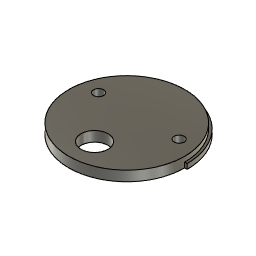
Bulkplate_InnerPayload_Cap_Subscale v1 (Autodesk Fusion 360 design; units mm, degrees)
Autodesk Fusion 360 part; units mm, degrees
sketch "Sketch1" plane through (0, 0, 0) normal (0, 0, 1) x (1, 0, 0)
  circle A0 centre (0, 0) radius 38.0746
  dimension "d1" = 76.1492
  constraint coincident A0.centre origin
  measures "d1" diameter of A0
extrude "Extrude1" add sketch "Sketch1" along normal blind 3.175
sketch "Sketch2" plane through (0, 0, 3.175) normal (0, 0, 1) x (-1, 0, 0)
  circle A0 centre (0, 0) radius 38.0746
  circle A1 centre (0, 0) radius 36.5125
  dimension "d4" = 73.025
  constraint concentric A0 A1
  measures "d4" diameter of A1
extrude "Extrude2" add sketch "Sketch2" along normal blind 3.175 contours A1
sketch "Sketch3" plane through (0, 0, 6.35) normal (0, 0, 1) x (-1, 0, 0)
  circle A0 centre (0, 0) radius 36.5125
  circle A1 centre (25.4, -7.62) radius 3.175
  circle A2 centre (-25.4, -7.62) radius 3.175
  circle A3 centre (0, 20.6756) radius 5.08
  circle A4 centre (0, 0) radius 38.0746
  dimension "d7" = 50.8
  dimension "d8" = 25.4
  dimension "d9" = 7.62
  dimension "d10" = 6.35
  dimension "d11" = 6.35
  dimension "d12" = 10.16
  dimension "d13" = 20.6756
  measures "d7" distance of A1.centre A2.centre
  measures "d8" horizontal distance of A0.centre A1.centre
  measures "d9" vertical distance of A0.centre A2.centre
  measures "d10" diameter of A2
  measures "d11" diameter of A1
  measures "d12" diameter of A3
  measures "d13" distance of A3.centre A0.centre
extrude "Extrude3" cut sketch "Sketch3" against normal blind 6.35 contours A1 | A2 | A3
sketch "Sketch4" plane through (0, 0, 6.35) normal (0, 0, 1) x (-1, 0, 0)
  circle A0 centre (-25.4, -7.62) radius 3.175
  circle A1 centre (0, 20.6756) radius 5.08
  circle A2 centre (25.4, -7.62) radius 3.175
  circle A3 centre (0, 0) radius 36.5125
  line L0 (38.0746, -0.0035) -> (36.5125, -0.0035)
  line L1 (-38.0746, 0.0019) -> (-36.5125, 0.0019)
  arc A4 (38.0746, -0.0035) -> (-38.0746, 0.0019) centre (0, 0) ccw
  arc A5 (36.5125, -0.0035) -> (-36.5125, 0.0019) centre (0, 0) ccw
  circle A6 centre (0, 20.6756) radius 8.509
  dimension "d16" = 76.1492
  dimension "d17" = 73.025
  dimension "d19" = 17.018
  constraint coincident A3.centre A4.centre
  constraint concentric A4 A5
  constraint horizontal L0
  constraint horizontal L1
  constraint concentric A1 A6
  measures "d16" diameter of A4
  measures "d17" diameter of A5
  measures "d19" diameter of A6
extrude "Extrude4" cut sketch "Sketch4" against normal through all contours A3 L0 L1 A4 A5
sketch "Sketch6" plane through (0, 0, 6.35) normal (0, 0, 1) x (1, 0, 0)
  circle A0 centre (0, -20.32) radius 8.509
  dimension "d20" = 17.018
  measures "d20" diameter of A0
extrude "Extrude5" cut sketch "Sketch6" against normal blind 27.94
equation "d2 = ( 0.25 / 2 ) * 1 in"
equation "d5 = ( 0.25 / 2 ) * 1 in"
